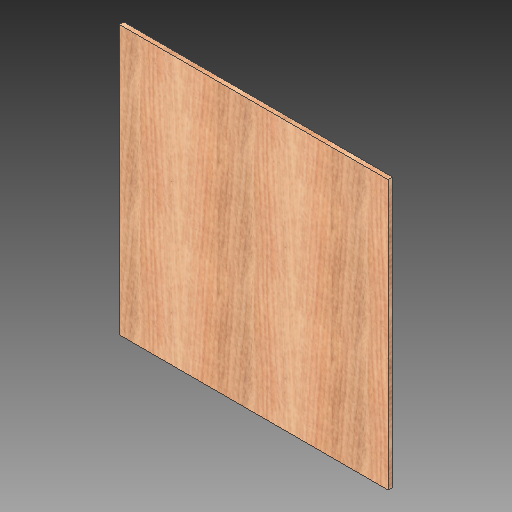
# Autodesk Inventor part: base1
Saved by Autodesk Inventor 2019 (Build 230136000, 136)
## iProperties
Created: 2019-01-07
Part Number: base1
Material: Wood (Birch)
Document SubType Name: Modeling
Designer: gaincarlo
Density: 0.55 g/cm^3
Appearance: Birch - Natural Polished
Project: La Panca - Flower Vase
Author: gaincarlo
Autodesk Inventor part; units mm, degrees
ref_plane "YZ Plane" through (0, 0, 0) normal (1, 0, 0) x (0, 1, 0)
ref_plane "XZ Plane" through (0, 0, 0) normal (0, 1, 0) x (-1, 0, 0)
ref_plane "Work Plane1" through (-212.7678, 7.004, 148.7409) normal (0, 0, 1) x (1, 0, 0)
sketch "Sketch1" plane through (-212.7678, 7.004, 148.7409) normal (0, 0, 1) x (1, 0, 0)
  line L0 (-178.2935, 300) -> (421.7065, 300)
  line L1 (421.7065, 300) -> (421.7065, -300)
  line L2 (421.7065, -300) -> (-178.2935, -300)
  line L3 (-178.2935, -300) -> (-178.2935, 300)
  line L4 (0, 0) -> (-339.8048, 0) construction
  arc A0 (-146.0745, -65.6505) -> (-145.6636, 64.6258) centre (-308.2935, 0) ccw construction
  point P0 (212.7678, -7.004)
  point P1 (-178.2935, 0)
  dimension "d0" = 600
  dimension "d1" = 600
  dimension "d2" = 130
  constraints: 10 end point, 2 horizontal, 2 parallel, 2 point on line, 1 midpoint, 1 perpendicular
  measures "d0" distance of L1.end L2.end
  measures "d1" distance of L0.end L1.end
  measures "d2" distance from line of L3 A0.centre
extrude "Extrusion1" add sketch "Sketch1" along normal blind 10
body "Solid1"
